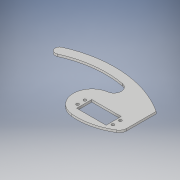
# Autodesk Inventor part: wstepna_geometria_wersja_2
Saved by Autodesk Inventor 2019 (Build 230136000, 136)
## iProperties
Created: 2022-02-09
Part Number: wstepna_geometria_wersja_2
Material: Generic
Document SubType Name: Modeling
Designer: Tomasz Krakowski
Density: 1 g/cm^3
Appearance: Default
Author: Tomasz Krakowski
Autodesk Inventor part; units mm, degrees
ref_plane "YZ Plane" through (0, 0, 0) normal (1, 0, 0) x (0, 1, 0)
ref_plane "XZ Plane" through (0, 0, 0) normal (0, 1, 0) x (-1, 0, 0)
ref_plane "XY Plane" through (0, 0, 0) normal (0, 0, 1) x (1, 0, 0)
sketch "Sketch1" plane through (0, 0, 0) normal (0, 1, 0) x (-1, 0, 0)
  arc A0 (-1.4142, 9.8995) -> (-10, 0) centre (0, 0) ccw
  line L0 (-39.5, 50.25) -> (0.5, 50.25)
  line L1 (0.5, 50.25) -> (0.5, 29.75)
  line L2 (0.5, 29.75) -> (-39.5, 29.75)
  line L3 (-39.5, 29.75) -> (-39.5, 50.25)
  line L4 (-39.5, 50.25) -> (0.5, 29.75) construction
  line L5 (0.5, 50.25) -> (-39.5, 29.75) construction
  line L6 (-10, 40) -> (-19.5, 40) construction
  circle A1 centre (4.5, 35) radius 1.9
  circle A2 centre (4.5, 45) radius 1.9
  line L7 (4.5, 45) -> (4.5, 35) construction
  circle A3 centre (-43.5, 45) radius 1.9
  circle A4 centre (-43.5, 35) radius 1.9
  line L8 (-43.5, 45) -> (-43.5, 35) construction
  line L9 (-43.5, 40) -> (-19.5, 40) construction
  line L10 (-10, 40) -> (4.5, 40) construction
  line L11 (-43.5, 45) -> (4.5, 45) construction
  line L12 (-43.5, 35) -> (4.5, 35) construction
  line L13 (-19.5, 40) -> (-19.5, 45) construction
  circle A5 centre (-10, 40) radius 9.75 construction
  circle A6 centre (-29, 40) radius 9.75 construction
  arc A7 (-2.7044, 60.2512) -> (-52.4397, 48.5007) centre (-10, -20) ccw
  arc A8 (-1.4142, 9.8995) -> (-2.7044, 60.2512) centre (-5, 35) ccw
  line L14 (-57.1731, 40) -> (-57.1731, 0)
  line L15 (-57.1731, 0) -> (0, 0) construction
  arc A9 (-52.4397, 48.5007) -> (-57.1731, 40) centre (-47.1731, 40) ccw
  line L16 (0, 0) -> (10, 0) construction
  line L17 (-10, 0) -> (-57.1731, 0) construction
  arc A10 (-10, 0) -> (-1.4142, -9.8995) centre (0, 0) ccw
  arc A11 (-1.8715, -9.8233) -> (77.546, -0.5248) centre (23.0596, 121.0399) ccw
  arc A12 (82.454, -11.4752) -> (77.546, -0.5248) centre (80, -6) ccw
  arc A13 (-57.1731, 0) -> (82.454, -11.4752) centre (23.0596, 121.0399) ccw
  line L18 (0, 0) -> (100, 0) construction
  point P0 (-57.1731, 45.3313)
  point P1 (-5, -35)
  dimension "d0" = 20
  dimension "d1" = 40
  dimension "d2" = 20.5
  dimension "d4" = 48
  dimension "d5" = 3.8
  dimension "d6" = 10
  dimension "d7" = 19.5
  dimension "d8" = 10
  dimension "d9" = 40
  dimension "d11" = 10.5
  dimension "d12" = 35
  dimension "d13" = 5
  dimension "d16" = 10
  dimension "d17" = 20
  dimension "d18" = 10
  dimension "d19" = 40
  dimension "d47" = 12
  dimension "d48" = 100
  dimension "d49" = 80
  dimension "d60" = 14.5
  constraints: 38 end point, 18 point on circle, 14 centre point, 8 tangent, 6 horizontal, 5 midpoint, 4 equal radius, 4 perpendicular, 3 coincident, 3 point on line, 2 collinear, 2 parallel, 2 symmetric about line, 2 vertical, 1 concentric, 1 other
  measures "d0" diameter of A0
  measures "d1" distance between parallel lines of L3 L1
  measures "d2" distance between parallel lines of L0 L2
  measures "d4" distance between parallel lines of L8 L7
  measures "d5" diameter of A1
  measures "d6" distance of L7.end L7.start
  measures "d7" diameter of A5
  measures "d8" horizontal distance of point (0, 0) L6.start
  measures "d9" vertical distance of point (0, 0) L6.start
  measures "d11" distance from line of L3 A6.centre
  measures "d12" vertical distance of point (0, 0) A8.centre
  measures "d13" horizontal distance of point (0, 0) A8.centre
  measures "d16" radius of A9
  measures "d17" vertical distance of point (0, 0) A7.centre
  measures "d18" horizontal distance of point (0, 0) A7.centre
  measures "d19" distance of L14.start L14.end
  measures "d47" diameter of A12
  measures "d48" distance of L18.end point (0, 0)
  measures "d49" horizontal distance of point (0, 0) A12.centre
  measures "d60" distance from line of A5.centre L7
extrude "Extrusion1" add sketch "Sketch1" along normal blind 3
equation "\"d11\" = d3"
equation "\"d3\" = 10.5"
body "Solid1"
